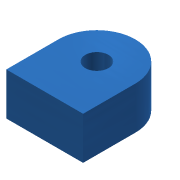
# Autodesk Inventor part: Current_transducer
Saved by Autodesk Inventor 2016 SP2 (Build 200236200, 236)
## iProperties
Created: 2017-09-22
Part Number: Current_transducer
Material: Generic
Document SubType Name: Modeling
Designer: Daan Giesen
Density: 0.001 g/cm^3
Appearance: Cyan
Project: Digital PID Loop
Cost Center: 17-0028
User Status: Work in Progress
Authority: Reichsöllner, Lukas
RuleStatus: InUse
Category: IOP
Company: Universiteit van Amsterdam
BeforeDocSave0: Open Form
Author: Daan Giesen
Title: Digital PID Loop
Revision Number: A
Autodesk Inventor part; units mm, degrees
ref_plane "YZ Plane" through (0, 0, 0) normal (1, 0, 0) x (0, 1, 0)
ref_plane "XZ Plane" through (0, 0, 0) normal (0, 1, 0) x (-1, 0, 0)
ref_plane "XY Plane" through (0, 0, 0) normal (0, 0, 1) x (1, 0, 0)
sketch "Sketch1" plane through (0, 0, 0) normal (0, 0, 1) x (1, 0, 0)
  line L0 (0, 73.4) -> (0, -97.4) construction
  line L1 (-68.6, 0) -> (68.6, 0) construction
  circle A0 centre (0, 0) radius 13
  arc A1 (49, 0) -> (-49, 0) centre (0, 0) ccw
  line L2 (-49, 0) -> (-49, -73)
  line L3 (-49, -73) -> (49, -73)
  line L4 (49, -73) -> (49, 0)
  dimension "d0" = 26
  dimension "d1" = 49
  dimension "d2" = 73
  constraints: 6 end point, 2 centre point, 2 coincident, 2 point on circle, 2 tangent, 1 horizontal, 1 parallel, 1 point on line
  measures "d0" diameter of A0
  measures "d1" radius of A1
  measures "d2" distance of L3.end L4.end
extrude "Extrusion1" add sketch "Sketch1" along normal mid plane 57
sketch "Sketch2" plane through (0, 0, -28.5) normal (0, 0, -1) x (-1, 0, 0)
  line L0 (-49, -73) -> (49, -73) projected
  point P0 (0, 0)
  point P1 (31, -48)
  point P2 (-31, -48)
  dimension "d5" = 31
  dimension "d6" = 31
  dimension "d7" = 25
  constraints: 1 horizontal alignment
  measures "d5" horizontal distance of point (0, 0) point (31, -48)
  measures "d6" horizontal distance of point (0, 0) point (-31, -48)
  measures "d7" distance from line of L0 point (31, -48)
hole "Hole1" at (-31, -48, -28.5) at (31, -48, -28.5) direction (0, 0, 1) diameter 4.917 depth 10 tip angle 118 thread size "M6x1" class "6H" standard "ISO Metric profile"
equation "\"d6\" = d5"
body "Solid1"
